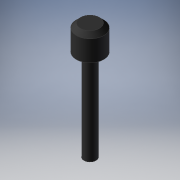
# Autodesk Inventor part: C-AC0806_r
Saved by Autodesk Inventor 2019 (Build 230136000, 136)
## iProperties
Created: 2023-10-14
Part Number: C-AC0806_r
Material: Generic
Catalog Web Link: www.cadenas.de
Description: C-AC-rod-C-VALUE Shock Absorbers - Double-stage Type
Vendor: MISUMI
Document SubType Name: Modeling
Designer: psAdmin
Manufacturer: MISUMI
Mass: 0.341266 g
Surface Area: 3.79817 cm^2
Volume: 0.341266 cm^3
Density: 1 g/cm^3
Appearance: PSOLRGB-175-175-175
Category: PARTsolutions
Company: MISUMI
Title: C-AC0806
Author: Cadenas PARTsolutions
Comments: C-VALUE Shock Absorbers - Double-stage Type
PSOL_IDENT_0: {$CADENAS_DATA/23d-libs/misumi/metric/29_springs/c_ac____/c_ac_____rod.prj},163 {VTYP=3D},{NB=C-AC08
PSOL_IDENT_1: 06_r},{LINA=C-AC0806},{NN=C-AC-rod},{DATE=28.09.2022 00:58:39},{GEOMDATE=19.05.2022 01:39:44},{VERSI
PSOL_IDENT_2: ON=},{LINEID=160},{WBVAR=TS},{WBNUMERIC=}  {NB=C-AC0806_r},{LINA=C-AC0806},{KT=DUMMY},{PN=C-AC0806},
PSOL_IDENT_3: {TYPE=C-AC0806},{TS=Cap},{TSALG= 'Cap','Cap','No Cap','No Cap' },{NO=0806},{S=6},{DD1=2.9},{L=16},{T
PSOL_IDENT_4: T=6.000},{DD=6.600},{TT1=1.000}
NB: C-AC0806_r
NN: C-AC-rod
NT: C-VALUE Shock Absorbers - Double-stage Type
NBSYN: $PN._r
LINA: C-AC0806
CATALOG: Misumi
PN: C-AC0806
NO: 0806
S: 6
DD1: 2.9
L: 16
SUPPLIER: MISUMI
ARTICLENO: C-AC0806_r
BOMINFO: C-AC0806
CREATOR: CADENAS GmbH
Autodesk Inventor part; units mm, degrees
sketch "Sketch_1" plane through (0, 0, 0) normal (0, 0, 1) x (1, 0, 0)
  line L0 (0, -22) -> (0, 0)
  line L1 (0, 0) -> (1.45, 0)
  line L2 (1.45, 0) -> (1.45, -22)
  line L3 (1.45, -22) -> (0, -22)
  line L4 (0, -22) -> (0, 0)
  constraints: 10 end point
revolve "Revolution1" add sketch "Sketch_1" angle 360 about axis through (0, -22, 0) along (0, -1, 0)
sketch "_____2" plane through (0, 0, 0) normal (0, 0, 1) x (1, 0, 0)
  line L0 (0, -50) -> (0, 50)
  line L1 (0, 6) -> (2.3, 6)
  line L2 (2.3, 6) -> (3.3, 5)
  line L3 (3.3, 5) -> (3.3, 0)
  line L4 (3.3, 0) -> (0, 0)
  line L5 (0, 0) -> (0, 6)
  constraints: 12 end point
revolve "Revolution2" add sketch "_____2" angle 360 about axis through (0, -50, 0) along (0, -1, 0)
ref_plane "to_body_XY" through (0, -6, 0) normal (0, -1, 0) x (1, 0, 0)
ref_plane "to_body_YZ" through (0, -6, 0) normal (1, 0, 0) x (0, 0, 1)
ref_plane "to_body_ZX" through (0, -6, 0) normal (0, 0, 1) x (0, -1, 0)
ref_plane "to_cap_XY" through (0, 0, 0) normal (0, -1, 0) x (1, 0, 0)
ref_plane "to_cap_YZ" through (0, 0, 0) normal (1, 0, 0) x (0, 0, 1)
ref_plane "to_cap_ZX" through (0, 0, 0) normal (0, 0, 1) x (0, -1, 0)
body "Solid1"
